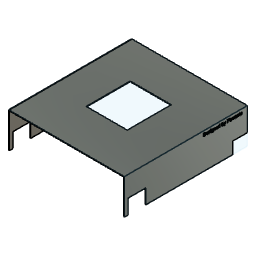
tapa horus v2 (Autodesk Fusion 360 design; units mm, degrees)
Autodesk Fusion 360 part; units mm, degrees
note: some values were not read from the file. Chosen so that the rebuilt part matches the saved one: which bodies a step acts on; which face or edge a step refers to.
sketch "Sketch1" plane through (0, 0, 0) normal (0, 0, 1) x (1, 0, 0)
  line L0 (0, 0) -> (395, 0)
  line L1 (395, 0) -> (395, 420)
  line L2 (395, 420) -> (0, 420)
  line L3 (0, 420) -> (0, 0)
  dimension "d1" = 395
  dimension "d2" = 420
  constraint horizontal L0
  constraint vertical L1
  constraint horizontal L2
  constraint vertical L3
  constraint coincident L0.start L3.end
  measures "d1" distance of L0.start L0.end
  measures "d2" distance of L0.start L2.end
extrude "Extrude1" add sketch "Sketch1" along normal blind 120 makes body 1
shell "Shell1" thickness 2 removed faces 1 at (131.6667, 280, 0) on bodies 1
sketch "Sketch2" plane through (0, 0, 120) normal (0, 0, 1) x (-1, 0, 0)
  line L0 (0, -420) -> (0, 0)
  line L1 (0, 0) -> (-395, 0)
  line L2 (-395, 0) -> (-395, -420)
  line L3 (-395, -420) -> (0, -420)
  line L4 (-262.5, -142.5) -> (-122.5, -142.5)
  line L5 (-122.5, -142.5) -> (-122.5, -292.5)
  line L6 (-122.5, -292.5) -> (-262.5, -292.5)
  line L7 (-262.5, -292.5) -> (-262.5, -142.5)
  line L8 (-262.5, -142.5) -> (-122.5, -292.5) construction
  line L9 (-122.5, -142.5) -> (-262.5, -292.5) construction
  point P0 (-192.5, -217.5)
  dimension "d6" = 140
  dimension "d7" = 150
  constraint horizontal L4
  constraint perpendicular L4 L5
  constraint parallel L4 L6
  constraint parallel L5 L7
  constraint coincident L8 P0
  constraint coincident L9 P0
  measures "d6" distance of L5.end L6.end
  measures "d7" distance of L4.end L5.end
extrude "Extrude2" cut sketch "Sketch2" against normal blind 50 contours L4 L5 L6 L7 bodies 1
sketch "Sketch3" plane through (0, 0, 120) normal (0, 0, 1) x (-1, 0, 0)
  line L0 (-122.5, -142.5) -> (-122.5, -292.5)
  line L1 (-122.5, -292.5) -> (-262.5, -292.5)
  line L2 (-262.5, -292.5) -> (-262.5, -142.5)
  line L3 (-262.5, -142.5) -> (-122.5, -142.5)
  line L4 (0, -420) -> (0, 0)
  line L5 (0, 0) -> (-395, 0)
  line L6 (-395, 0) -> (-395, -420)
  line L7 (-395, -420) -> (0, -420)
  dimension "d10" = 420
  measures "d10" distance of L4.start L5
sketch "Sketch4" plane through (395, 0, 0) normal (1, 0, 0) x (0, 1, 0)
  line L0 (0, 0) -> (420, 0)
  line L1 (420, 0) -> (420, 120)
  line L2 (420, 120) -> (0, 120)
  line L3 (0, 120) -> (0, 0)
  line L4 (0, 0) -> (13, 0)
  line L5 (13, 0) -> (73, 0)
  line L6 (73, 0) -> (73, 50)
  line L7 (73, 50) -> (13, 50)
  line L8 (13, 50) -> (13, 0)
  dimension "d11" = 13
  dimension "d12" = 60
  dimension "d13" = 50
  constraint coincident L0.start L3.end
  constraint perpendicular L3 L4
  constraint horizontal L5
  constraint vertical L6
  constraint horizontal L7
  constraint vertical L8
  measures "d11" distance of L0.start L4.end
  measures "d12" distance of L4.end L5.end
  measures "d13" distance of L4.end L7.end
extrude "Extrude3" cut sketch "Sketch4" against normal blind 600 contours L0 L5 L6 L7 L8 bodies 1
sketch "Sketch5" plane through (395, 0, 0) normal (1, 0, 0) x (0, 1, 0)
  line L0 (13, 0) -> (13, 50)
  line L1 (13, 50) -> (73, 50)
  line L2 (73, 50) -> (73, 0)
  line L3 (73, 0) -> (420, 0)
  line L4 (420, 0) -> (420, 120)
  line L5 (420, 120) -> (0, 120)
  line L6 (0, 120) -> (0, 0)
  line L7 (0, 0) -> (13, 0)
extrude "Extrude4" cut 1 faces at (132.3333, 2, 78.6667) along direction (0, -1, 0) blind 80 on bodies 1 bodies 1
sketch "Sketch6" plane through (395, 0, 0) normal (1, 0, 0) x (0, 1, 0)
  line L0 (270.0115, 67.3686) -> (420.0115, 67.3686) construction
  line L1 (420.0115, 67.3686) -> (420.0115, 112.709) construction
  line L2 (420.0115, 112.709) -> (270.0115, 112.709) construction
  line L3 (270.0115, 112.709) -> (270.0115, 67.3686) construction
  dimension "d18" = 10
  text T0 "Designed by Ferrante" font "Arial" height 10 align left top in box 150 x 45.3404 at (270.0115, 67.3686) x (1, 0) y (0, 1) spacing 1
extrude "Extrude5" cut sketch "Sketch6" against normal blind 100 text T0 bodies 1 makes body 2 at (393, 274.6067, 107.734) makes body 3 at (395, 323.4069, 108.1486) makes body 4 at (395, 335.189, 105.9572) makes body 5 at (395, 380.4941, 105.4237) makes body 6 at (394.3333, 362.2056, 107.0269) makes body 7 at (394.3333, 398.6995, 107.0269) makes body 8 at (394.3333, 315.6163, 107.0269) makes body 9 at (395, 301.0213, 104.6144) makes body 10 at (219.1667, 47.5, 120)
sketch "Sketch7" plane through (395, 0, 0) normal (1, 0, 0) x (0, 1, 0)
  line L0 (420, 0) -> (370, 0)
  line L1 (370, 0) -> (370, 40)
  line L2 (370, 40) -> (420, 40)
  line L3 (420, 40) -> (420, 0)
  dimension "d21" = 50
  dimension "d22" = 40
  constraint horizontal L0
  constraint vertical L1
  constraint horizontal L2
  constraint vertical L3
  measures "d21" distance of L0.start L0.end
  measures "d22" distance of L0.start L2.end
extrude "Extrude6" cut sketch "Sketch7" against normal blind 425 bodies 10
extrude "Extrude7" cut 1 faces at (262.6667, 418, 66) along direction (0, 1, 0) blind 175 on bodies 10 bodies 10
